Autodesk Inventor part; units mm, degrees
(part 2 of 2)
  line L838 (-99.3571, 77.0912) -> (-99.3571, 73.3912)
  line L839 (-99.3571, 73.3912) -> (-93.3571, 73.3912)
  line L840 (-93.3571, 73.3912) -> (-93.3571, 74.7912)
  line L841 (-91.3571, 74.7912) -> (-91.3571, 73.3912)
  line L842 (-91.3571, 73.3912) -> (-85.3571, 73.3912)
  line L843 (-85.3571, 73.3912) -> (-85.3571, 77.0912)
  line L844 (-85.3571, 77.0912) -> (-86.3571, 77.0912)
  line L845 (-86.3571, 77.0912) -> (-86.3571, 81.0912)
  spline S16 degree 3 poles (-86.3571, 81.0912) (-86.3571, 81.3565) (-86.4624, 81.6108) (-86.6499, 81.7984) knots 0 0 0 0 0.5 0.5 0.5 0.5
  line L846 (-86.3571, 81.0912) -> (-86.3571, 81.3565) construction
  line L847 (-86.3571, 81.3565) -> (-86.4624, 81.6108) construction
  line L848 (-86.4624, 81.6108) -> (-86.6499, 81.7984) construction
  spline S17 degree 3 poles (-86.6499, 81.7984) (-86.6501, 81.7986) (-86.8375, 81.9859) (-87.0918, 82.0912) (-87.3571, 82.0912) knots 0.5 0.5 0.5 0.5 0.5 1 1 1 1
  line L849 (-86.6499, 81.7984) -> (-86.6499, 81.7984) construction
  line L850 (-86.6499, 81.7984) -> (-86.8375, 81.9859) construction
  line L851 (-86.8375, 81.9859) -> (-87.0918, 82.0912) construction
  line L852 (-87.0918, 82.0912) -> (-87.3571, 82.0912) construction
  line L853 (-87.3571, 82.0912) -> (-89.3571, 82.0912)
  spline S18 degree 3 poles (-89.3571, 82.0912) (-89.6223, 82.0912) (-89.8766, 81.9859) (-90.0642, 81.7984) knots 0 0 0 0 0.5 0.5 0.5 0.5
  line L854 (-89.3571, 82.0912) -> (-89.6223, 82.0912) construction
  line L855 (-89.6223, 82.0912) -> (-89.8766, 81.9859) construction
  line L856 (-89.8766, 81.9859) -> (-90.0642, 81.7984) construction
  spline S19 degree 3 poles (-90.0642, 81.7984) (-90.0644, 81.7982) (-90.2517, 81.6108) (-90.3571, 81.3565) (-90.3571, 81.0912) knots 0.5 0.5 0.5 0.5 0.5 1 1 1 1
  line L857 (-90.0642, 81.7984) -> (-90.0642, 81.7984) construction
  line L858 (-90.0642, 81.7984) -> (-90.2517, 81.6108) construction
  line L859 (-90.2517, 81.6108) -> (-90.3571, 81.3565) construction
  line L860 (-90.3571, 81.3565) -> (-90.3571, 81.0912) construction
  line L861 (-90.3571, 81.0912) -> (-90.3571, 77.0912)
  line L862 (-90.3571, 77.0912) -> (-91.3571, 77.0912)
  line L863 (-91.3571, 77.0912) -> (-91.3571, 75.0912)
  line L864 (-91.3571, 91.7912) -> (-91.3571, 90.3912)
  line L865 (-91.3571, 90.3912) -> (-85.3571, 90.3912)
  line L866 (-85.3571, 90.3912) -> (-85.3571, 94.0912)
  line L867 (-85.3571, 94.0912) -> (-86.3571, 94.0912)
  line L868 (-86.3571, 94.0912) -> (-86.3571, 98.0911)
  spline S20 degree 3 poles (-86.3571, 98.0911) (-86.3571, 98.3564) (-86.4624, 98.6107) (-86.6499, 98.7983) knots 0 0 0 0 0.5 0.5 0.5 0.5
  line L869 (-86.3571, 98.0911) -> (-86.3571, 98.3564) construction
  line L870 (-86.3571, 98.3564) -> (-86.4624, 98.6107) construction
  line L871 (-86.4624, 98.6107) -> (-86.6499, 98.7983) construction
  spline S21 degree 3 poles (-86.6499, 98.7983) (-86.6501, 98.7985) (-86.8375, 98.9858) (-87.0918, 99.0911) (-87.3571, 99.0911) knots 0.5 0.5 0.5 0.5 0.5 1 1 1 1
  line L872 (-86.6499, 98.7983) -> (-86.6499, 98.7983) construction
  line L873 (-86.6499, 98.7983) -> (-86.8375, 98.9858) construction
  line L874 (-86.8375, 98.9858) -> (-87.0918, 99.0911) construction
  line L875 (-87.0918, 99.0911) -> (-87.3571, 99.0911) construction
  line L876 (-87.3571, 99.0911) -> (-89.3571, 99.0911)
  spline S22 degree 3 poles (-89.3571, 99.0911) (-89.6223, 99.0911) (-89.8766, 98.9858) (-90.0642, 98.7983) knots 0 0 0 0 0.5 0.5 0.5 0.5
  line L877 (-89.3571, 99.0911) -> (-89.6223, 99.0911) construction
  line L878 (-89.6223, 99.0911) -> (-89.8766, 98.9858) construction
  line L879 (-89.8766, 98.9858) -> (-90.0642, 98.7983) construction
  spline S23 degree 3 poles (-90.0642, 98.7983) (-90.0644, 98.7981) (-90.2517, 98.6107) (-90.3571, 98.3564) (-90.3571, 98.0911) knots 0.5 0.5 0.5 0.5 0.5 1 1 1 1
  line L880 (-90.0642, 98.7983) -> (-90.0642, 98.7983) construction
  line L881 (-90.0642, 98.7983) -> (-90.2517, 98.6107) construction
  line L882 (-90.2517, 98.6107) -> (-90.3571, 98.3564) construction
  line L883 (-90.3571, 98.3564) -> (-90.3571, 98.0911) construction
  line L884 (-90.3571, 98.0911) -> (-90.3571, 94.0912)
  line L885 (-90.3571, 94.0912) -> (-91.3571, 94.0912)
  line L886 (-91.3571, 94.0912) -> (-91.3571, 92.0912)
  line L887 (-93.3571, 92.0912) -> (-93.3571, 94.0912)
  line L888 (-93.3571, 94.0912) -> (-94.3571, 94.0912)
  line L889 (-94.3571, 94.0912) -> (-94.3571, 98.0911)
  spline S24 degree 3 poles (-94.3571, 98.0911) (-94.3571, 98.3564) (-94.4624, 98.6107) (-94.6499, 98.7983) knots 0 0 0 0 0.5 0.5 0.5 0.5
  line L890 (-94.3571, 98.0911) -> (-94.3571, 98.3564) construction
  line L891 (-94.3571, 98.3564) -> (-94.4624, 98.6107) construction
  line L892 (-94.4624, 98.6107) -> (-94.6499, 98.7983) construction
  spline S25 degree 3 poles (-94.6499, 98.7983) (-94.6501, 98.7985) (-94.8375, 98.9858) (-95.0918, 99.0911) (-95.3571, 99.0911) knots 0.5 0.5 0.5 0.5 0.5 1 1 1 1
  line L893 (-94.6499, 98.7983) -> (-94.6499, 98.7983) construction
  line L894 (-94.6499, 98.7983) -> (-94.8375, 98.9858) construction
  line L895 (-94.8375, 98.9858) -> (-95.0918, 99.0911) construction
  line L896 (-95.0918, 99.0911) -> (-95.3571, 99.0911) construction
  line L897 (-95.3571, 99.0911) -> (-97.3571, 99.0911)
  spline S26 degree 3 poles (-97.3571, 99.0911) (-97.6223, 99.0911) (-97.8766, 98.9858) (-98.0642, 98.7983) knots 0 0 0 0 0.5 0.5 0.5 0.5
  line L898 (-97.3571, 99.0911) -> (-97.6223, 99.0911) construction
  line L899 (-97.6223, 99.0911) -> (-97.8766, 98.9858) construction
  line L900 (-97.8766, 98.9858) -> (-98.0642, 98.7983) construction
  spline S27 degree 3 poles (-98.0642, 98.7983) (-98.0644, 98.7981) (-98.2517, 98.6107) (-98.3571, 98.3564) (-98.3571, 98.0911) knots 0.5 0.5 0.5 0.5 0.5 1 1 1 1
  line L901 (-98.0642, 98.7983) -> (-98.0642, 98.7983) construction
  line L902 (-98.0642, 98.7983) -> (-98.2517, 98.6107) construction
  line L903 (-98.2517, 98.6107) -> (-98.3571, 98.3564) construction
  line L904 (-98.3571, 98.3564) -> (-98.3571, 98.0911) construction
  line L905 (-98.3571, 98.0911) -> (-98.3571, 94.0912)
  line L906 (-98.3571, 94.0912) -> (-99.3571, 94.0912)
  line L907 (-99.3571, 94.0912) -> (-99.3571, 90.3912)
  line L908 (-99.3571, 90.3912) -> (-93.3571, 90.3912)
  line L909 (-93.3571, 90.3912) -> (-93.3571, 91.7912)
  line L910 (-93.3571, 91.7912) -> (-91.3571, 91.7912)
  line L911 (-91.3571, 92.0912) -> (-93.3571, 92.0912)
  line L912 (-38.6965, 73.0892) -> (-34.6965, 73.0892)
  line L913 (-34.6965, 73.0892) -> (-34.6965, 76.0892)
  line L914 (-34.6965, 76.0892) -> (-38.6965, 76.0892)
  line L915 (-38.6965, 76.0892) -> (-38.6965, 73.0892)
  line L916 (-93.2175, 103.1942) -> (-89.2175, 103.1942)
  line L917 (-89.2175, 103.1942) -> (-89.2175, 106.1942)
  line L918 (-89.2175, 106.1942) -> (-93.2175, 106.1942)
  line L919 (-93.2175, 106.1942) -> (-93.2175, 103.1942)
  line L920 (-93.2175, 110.1942) -> (-89.2175, 110.1942)
  line L921 (-89.2175, 110.1942) -> (-89.2175, 113.1942)
  line L922 (-89.2175, 113.1942) -> (-93.2175, 113.1942)
  line L923 (-93.2175, 113.1942) -> (-93.2175, 110.1942)
  line L924 (73.6427, 117.4429) -> (68.6427, 117.4429)
  line L925 (68.6427, 117.4429) -> (68.6427, 120.4429)
  line L926 (68.6427, 120.4429) -> (73.6427, 120.4429)
  line L927 (73.6427, 120.4429) -> (73.6427, 117.4429)
  line L928 (73.6427, 58.7395) -> (68.6427, 58.7395)
  line L929 (68.6427, 58.7395) -> (68.6427, 55.7395)
  line L930 (68.6427, 55.7395) -> (73.6427, 55.7395)
  line L931 (73.6427, 55.7395) -> (73.6427, 58.7395)
  line L932 (-93.1735, 117.4429) -> (-88.1735, 117.4429)
  line L933 (-88.1735, 117.4429) -> (-88.1735, 120.4429)
  line L934 (-88.1735, 120.4429) -> (-93.1735, 120.4429)
  line L935 (-93.1735, 120.4429) -> (-93.1735, 117.4429)
  spline S28 degree 3 poles (-84.0914, 112.2529) (-84.0914, 113.0813) (-84.763, 113.7529) (-85.5914, 113.7529) knots 0 0 0 0 0.25 0.25 0.25 0.25
  line L936 (-84.0914, 112.2529) -> (-84.0914, 113.0813) construction
  line L937 (-84.0914, 113.0813) -> (-84.763, 113.7529) construction
  line L938 (-84.763, 113.7529) -> (-85.5914, 113.7529) construction
  line L939 (-85.5914, 113.7529) -> (-85.5914, 113.7529) construction
  line L940 (-85.5914, 113.7529) -> (-86.4199, 113.7529) construction
  line L941 (-86.4199, 113.7529) -> (-87.0914, 113.0813) construction
  line L942 (-87.0914, 113.0813) -> (-87.0914, 112.2529) construction
  line L943 (-87.0914, 112.2529) -> (-87.0914, 112.2529) construction
  line L944 (-87.0914, 112.2529) -> (-87.0914, 111.4245) construction
  line L945 (-87.0914, 111.4245) -> (-86.4199, 110.7529) construction
  line L946 (-86.4199, 110.7529) -> (-85.5914, 110.7529) construction
  line L947 (-85.5914, 110.7529) -> (-85.5914, 110.7529) construction
  line L948 (-85.5914, 110.7529) -> (-84.763, 110.7529) construction
  line L949 (-84.763, 110.7529) -> (-84.0914, 111.4245) construction
  line L950 (-84.0914, 111.4245) -> (-84.0914, 112.2529) construction
  spline S29 degree 3 poles (-84.0914, 63.993) (-84.0914, 64.8214) (-84.763, 65.493) (-85.5914, 65.493) knots 0 0 0 0 0.25 0.25 0.25 0.25
  line L951 (-84.0914, 63.993) -> (-84.0914, 64.8214) construction
  line L952 (-84.0914, 64.8214) -> (-84.763, 65.493) construction
  line L953 (-84.763, 65.493) -> (-85.5914, 65.493) construction
  line L954 (-85.5914, 65.493) -> (-85.5914, 65.493) construction
  line L955 (-85.5914, 65.493) -> (-86.4199, 65.493) construction
  line L956 (-86.4199, 65.493) -> (-87.0914, 64.8214) construction
  line L957 (-87.0914, 64.8214) -> (-87.0914, 63.993) construction
  line L958 (-87.0914, 63.993) -> (-87.0914, 63.993) construction
  line L959 (-87.0914, 63.993) -> (-87.0914, 63.1646) construction
  line L960 (-87.0914, 63.1646) -> (-86.4199, 62.493) construction
  line L961 (-86.4199, 62.493) -> (-85.5914, 62.493) construction
  line L962 (-85.5914, 62.493) -> (-85.5914, 62.493) construction
  line L963 (-85.5914, 62.493) -> (-84.763, 62.493) construction
  line L964 (-84.763, 62.493) -> (-84.0914, 63.1646) construction
  line L965 (-84.0914, 63.1646) -> (-84.0914, 63.993) construction
  spline S30 degree 3 poles (-18.0514, 67.168) (-18.0514, 67.9964) (-18.723, 68.668) (-19.5514, 68.668) knots 0 0 0 0 0.25 0.25 0.25 0.25
  line L966 (-18.0514, 67.168) -> (-18.0514, 67.9964) construction
  line L967 (-18.0514, 67.9964) -> (-18.723, 68.668) construction
  line L968 (-18.723, 68.668) -> (-19.5514, 68.668) construction
  line L969 (-19.5514, 68.668) -> (-19.5514, 68.668) construction
  line L970 (-19.5514, 68.668) -> (-20.3799, 68.668) construction
  line L971 (-20.3799, 68.668) -> (-21.0514, 67.9964) construction
  line L972 (-21.0514, 67.9964) -> (-21.0514, 67.168) construction
  line L973 (-21.0514, 67.168) -> (-21.0514, 67.168) construction
  line L974 (-21.0514, 67.168) -> (-21.0514, 66.3396) construction
  line L975 (-21.0514, 66.3396) -> (-20.3799, 65.668) construction
  line L976 (-20.3799, 65.668) -> (-19.5514, 65.668) construction
  line L977 (-19.5514, 65.668) -> (-19.5514, 65.668) construction
  line L978 (-19.5514, 65.668) -> (-18.723, 65.668) construction
  line L979 (-18.723, 65.668) -> (-18.0514, 66.3396) construction
  line L980 (-18.0514, 66.3396) -> (-18.0514, 67.168) construction
  line L981 (-100.3571, 66.5242) -> (-100.3571, 55.7396)
  line L982 (-100.3571, 55.7395) -> (-100.3553, 55.6371)
  line L983 (-100.3553, 55.6371) -> (-100.3501, 55.5348)
  line L984 (-100.3501, 55.5348) -> (-100.3413, 55.4327)
  line L985 (-100.3413, 55.4327) -> (-100.3291, 55.331)
  line L986 (-100.3291, 55.331) -> (-100.3134, 55.2298)
  line L987 (-100.3134, 55.2298) -> (-100.2943, 55.1291)
  line L988 (-100.2943, 55.1291) -> (-100.2718, 55.0292)
  line L989 (-100.2718, 55.0292) -> (-100.2458, 54.9301)
  line L990 (-100.2458, 54.9301) -> (-100.2165, 54.832)
  line L991 (-100.2165, 54.832) -> (-100.1838, 54.7349)
  line L992 (-100.1838, 54.7349) -> (-100.1479, 54.6389)
  line L993 (-100.1479, 54.6389) -> (-100.1087, 54.5443)
  line L994 (-100.1087, 54.5443) -> (-100.0663, 54.451)
  line L995 (-100.0663, 54.451) -> (-100.0207, 54.3593)
  line L996 (-100.0207, 54.3593) -> (-99.972, 54.2692)
  line L997 (-99.972, 54.2692) -> (-99.9203, 54.1807)
  line L998 (-99.9203, 54.1807) -> (-99.8656, 54.0941)
  line L999 (-99.8656, 54.0941) -> (-99.808, 54.0095)
  line L1000 (-99.808, 54.0095) -> (-99.7475, 53.9268)
  line L1001 (-99.7475, 53.9268) -> (-99.6842, 53.8462)
  line L1002 (-99.6842, 53.8462) -> (-99.6182, 53.7679)
  line L1003 (-99.6182, 53.7679) -> (-99.5496, 53.6918)
  line L1004 (-99.5496, 53.6918) -> (-99.4784, 53.6182)
  line L1005 (-99.4784, 53.6182) -> (-99.4047, 53.547)
  line L1006 (-99.4047, 53.547) -> (-99.3287, 53.4784)
  line L1007 (-99.3287, 53.4784) -> (-99.2503, 53.4124)
  line L1008 (-99.2503, 53.4124) -> (-99.1698, 53.3491)
  line L1009 (-99.1698, 53.3491) -> (-99.0871, 53.2886)
  line L1010 (-99.0871, 53.2886) -> (-99.0024, 53.231)
  line L1011 (-99.0024, 53.231) -> (-98.9158, 53.1762)
  line L1012 (-98.9158, 53.1762) -> (-98.8274, 53.1245)
  line L1013 (-98.8274, 53.1245) -> (-98.7372, 53.0758)
  line L1014 (-98.7372, 53.0758) -> (-98.6455, 53.0303)
  line L1015 (-98.6455, 53.0303) -> (-98.5523, 52.9879)
  line L1016 (-98.5523, 52.9879) -> (-98.4576, 52.9487)
  line L1017 (-98.4576, 52.9487) -> (-98.3617, 52.9127)
  line L1018 (-98.3617, 52.9127) -> (-98.2646, 52.8801)
  line L1019 (-98.2646, 52.8801) -> (-98.1664, 52.8507)
  line L1020 (-98.1664, 52.8507) -> (-98.0673, 52.8248)
  line L1021 (-98.0673, 52.8248) -> (-97.9674, 52.8022)
  line L1022 (-97.9674, 52.8022) -> (-97.8668, 52.7831)
  line L1023 (-97.8668, 52.7831) -> (-97.7655, 52.7674)
  line L1024 (-97.7655, 52.7674) -> (-97.6638, 52.7552)
  line L1025 (-97.6638, 52.7552) -> (-97.5618, 52.7465)
  line L1026 (-97.5618, 52.7465) -> (-97.4595, 52.7412)
  line L1027 (-97.4595, 52.7412) -> (-97.3571, 52.7395)
  line L1028 (-97.3571, 52.7395) -> (-16.3571, 52.7395)
  line L1029 (-16.3571, 52.7395) -> (-16.2546, 52.7412)
  line L1030 (-16.2546, 52.7412) -> (-16.1523, 52.7465)
  line L1031 (-16.1523, 52.7465) -> (-16.0503, 52.7552)
  line L1032 (-16.0503, 52.7552) -> (-15.9486, 52.7674)
  line L1033 (-15.9486, 52.7674) -> (-15.8473, 52.7831)
  line L1034 (-15.8473, 52.7831) -> (-15.7467, 52.8022)
  line L1035 (-15.7467, 52.8022) -> (-15.6468, 52.8248)
  line L1036 (-15.6468, 52.8248) -> (-15.5477, 52.8507)
  line L1037 (-15.5477, 52.8507) -> (-15.4495, 52.8801)
  line L1038 (-15.4495, 52.8801) -> (-15.3524, 52.9127)
  line L1039 (-15.3524, 52.9127) -> (-15.2565, 52.9487)
  line L1040 (-15.2565, 52.9487) -> (-15.1618, 52.9879)
  line L1041 (-15.1618, 52.9879) -> (-15.0686, 53.0303)
  line L1042 (-15.0686, 53.0303) -> (-14.9769, 53.0758)
  line L1043 (-14.9769, 53.0758) -> (-14.8867, 53.1245)
  line L1044 (-14.8867, 53.1245) -> (-14.7983, 53.1762)
  line L1045 (-14.7983, 53.1762) -> (-14.7117, 53.231)
  line L1046 (-14.7117, 53.231) -> (-14.627, 53.2886)
  line L1047 (-14.627, 53.2886) -> (-14.5443, 53.3491)
  line L1048 (-14.5443, 53.3491) -> (-14.4638, 53.4124)
  line L1049 (-14.4638, 53.4124) -> (-14.3854, 53.4784)
  line L1050 (-14.3854, 53.4784) -> (-14.3094, 53.547)
  line L1051 (-14.3094, 53.547) -> (-14.2357, 53.6182)
  line L1052 (-14.2357, 53.6182) -> (-14.1645, 53.6918)
  line L1053 (-14.1645, 53.6918) -> (-14.0959, 53.7679)
  line L1054 (-14.0959, 53.7679) -> (-14.0299, 53.8462)
  line L1055 (-14.0299, 53.8462) -> (-13.9666, 53.9268)
  line L1056 (-13.9666, 53.9268) -> (-13.9061, 54.0095)
  line L1057 (-13.9061, 54.0095) -> (-13.8485, 54.0941)
  line L1058 (-13.8485, 54.0941) -> (-13.7938, 54.1807)
  line L1059 (-13.7938, 54.1807) -> (-13.7421, 54.2692)
  line L1060 (-13.7421, 54.2692) -> (-13.6934, 54.3593)
  line L1061 (-13.6934, 54.3593) -> (-13.6478, 54.451)
  line L1062 (-13.6478, 54.451) -> (-13.6054, 54.5443)
  line L1063 (-13.6054, 54.5443) -> (-13.5662, 54.6389)
  line L1064 (-13.5662, 54.6389) -> (-13.5303, 54.7349)
  line L1065 (-13.5303, 54.7349) -> (-13.4976, 54.832)
  line L1066 (-13.4976, 54.832) -> (-13.4683, 54.9301)
  line L1067 (-13.4683, 54.9301) -> (-13.4423, 55.0292)
  line L1068 (-13.4423, 55.0292) -> (-13.4198, 55.1291)
  line L1069 (-13.4198, 55.1291) -> (-13.4007, 55.2298)
  line L1070 (-13.4007, 55.2298) -> (-13.385, 55.331)
  line L1071 (-13.385, 55.331) -> (-13.3728, 55.4327)
  line L1072 (-13.3728, 55.4327) -> (-13.364, 55.5348)
  line L1073 (-13.364, 55.5348) -> (-13.3588, 55.6371)
  line L1074 (-13.3588, 55.6371) -> (-13.3571, 55.7395)
  line L1075 (-13.3571, 55.7395) -> (-13.3571, 120.4429)
  line L1076 (-13.3571, 120.4429) -> (-13.3588, 120.5453)
  line L1077 (-13.3588, 120.5453) -> (-13.364, 120.6476)
  line L1078 (-13.364, 120.6476) -> (-13.3728, 120.7497)
  line L1079 (-13.3728, 120.7497) -> (-13.385, 120.8514)
  line L1080 (-13.385, 120.8514) -> (-13.4007, 120.9526)
  line L1081 (-13.4007, 120.9526) -> (-13.4198, 121.0533)
  line L1082 (-13.4198, 121.0533) -> (-13.4423, 121.1532)
  line L1083 (-13.4423, 121.1532) -> (-13.4683, 121.2523)
  line L1084 (-13.4683, 121.2523) -> (-13.4976, 121.3504)
  line L1085 (-13.4976, 121.3504) -> (-13.5303, 121.4475)
  line L1086 (-13.5303, 121.4475) -> (-13.5662, 121.5435)
  line L1087 (-13.5662, 121.5435) -> (-13.6054, 121.6381)
  line L1088 (-13.6054, 121.6381) -> (-13.6478, 121.7314)
  line L1089 (-13.6478, 121.7314) -> (-13.6934, 121.8231)
  line L1090 (-13.6934, 121.8231) -> (-13.7421, 121.9132)
  line L1091 (-13.7421, 121.9132) -> (-13.7938, 122.0017)
  line L1092 (-13.7938, 122.0017) -> (-13.8485, 122.0883)
  line L1093 (-13.8485, 122.0883) -> (-13.9061, 122.1729)
  line L1094 (-13.9061, 122.1729) -> (-13.9666, 122.2556)
  line L1095 (-13.9666, 122.2556) -> (-14.0299, 122.3362)
  line L1096 (-14.0299, 122.3362) -> (-14.0959, 122.4145)
  line L1097 (-14.0959, 122.4145) -> (-14.1645, 122.4906)
  line L1098 (-14.1645, 122.4906) -> (-14.2357, 122.5642)
  line L1099 (-14.2357, 122.5642) -> (-14.3094, 122.6354)
  line L1100 (-14.3094, 122.6354) -> (-14.3854, 122.704)
  line L1101 (-14.3854, 122.704) -> (-14.4638, 122.77)
  line L1102 (-14.4638, 122.77) -> (-14.5443, 122.8333)
  line L1103 (-14.5443, 122.8333) -> (-14.627, 122.8938)
  line L1104 (-14.627, 122.8938) -> (-14.7117, 122.9514)
  line L1105 (-14.7117, 122.9514) -> (-14.7983, 123.0062)
  line L1106 (-14.7983, 123.0062) -> (-14.8867, 123.0579)
  line L1107 (-14.8867, 123.0579) -> (-14.9769, 123.1066)
  line L1108 (-14.9769, 123.1066) -> (-15.0686, 123.1521)
  line L1109 (-15.0686, 123.1521) -> (-15.1618, 123.1945)
  line L1110 (-15.1618, 123.1945) -> (-15.2565, 123.2337)
  line L1111 (-15.2565, 123.2337) -> (-15.3524, 123.2697)
  line L1112 (-15.3524, 123.2697) -> (-15.4495, 123.3023)
  line L1113 (-15.4495, 123.3023) -> (-15.5477, 123.3317)
  line L1114 (-15.5477, 123.3317) -> (-15.6468, 123.3576)
  line L1115 (-15.6468, 123.3576) -> (-15.7467, 123.3802)
  line L1116 (-15.7467, 123.3802) -> (-15.8473, 123.3993)
  line L1117 (-15.8473, 123.3993) -> (-15.9486, 123.415)
  line L1118 (-15.9486, 123.415) -> (-16.0503, 123.4272)
  line L1119 (-16.0503, 123.4272) -> (-16.1523, 123.4359)
  line L1120 (-16.1523, 123.4359) -> (-16.2546, 123.4412)
  line L1121 (-16.2546, 123.4412) -> (-16.3571, 123.4429)
  line L1122 (-16.3571, 123.4429) -> (-97.3571, 123.4429)
  line L1123 (-97.3571, 123.4429) -> (-97.4595, 123.4412)
  line L1124 (-97.4595, 123.4412) -> (-97.5618, 123.4359)
  line L1125 (-97.5618, 123.4359) -> (-97.6638, 123.4272)
  line L1126 (-97.6638, 123.4272) -> (-97.7655, 123.415)
  line L1127 (-97.7655, 123.415) -> (-97.8668, 123.3993)
  line L1128 (-97.8668, 123.3993) -> (-97.9674, 123.3802)
  line L1129 (-97.9674, 123.3802) -> (-98.0673, 123.3576)
  line L1130 (-98.0673, 123.3576) -> (-98.1664, 123.3317)
  line L1131 (-98.1664, 123.3317) -> (-98.2646, 123.3023)
  line L1132 (-98.2646, 123.3023) -> (-98.3617, 123.2697)
  line L1133 (-98.3617, 123.2697) -> (-98.4576, 123.2337)
  line L1134 (-98.4576, 123.2337) -> (-98.5523, 123.1945)
  line L1135 (-98.5523, 123.1945) -> (-98.6455, 123.1521)
  line L1136 (-98.6455, 123.1521) -> (-98.7372, 123.1066)
  line L1137 (-98.7372, 123.1066) -> (-98.8274, 123.0579)
  line L1138 (-98.8274, 123.0579) -> (-98.9158, 123.0062)
  line L1139 (-98.9158, 123.0062) -> (-99.0024, 122.9514)
  line L1140 (-99.0024, 122.9514) -> (-99.0871, 122.8938)
  line L1141 (-99.0871, 122.8938) -> (-99.1698, 122.8333)
  line L1142 (-99.1698, 122.8333) -> (-99.2503, 122.77)
  line L1143 (-99.2503, 122.77) -> (-99.3287, 122.704)
  line L1144 (-99.3287, 122.704) -> (-99.4047, 122.6354)
  line L1145 (-99.4047, 122.6354) -> (-99.4784, 122.5642)
  line L1146 (-99.4784, 122.5642) -> (-99.5496, 122.4906)
  line L1147 (-99.5496, 122.4906) -> (-99.6182, 122.4145)
  line L1148 (-99.6182, 122.4145) -> (-99.6842, 122.3362)
  line L1149 (-99.6842, 122.3362) -> (-99.7475, 122.2556)
  line L1150 (-99.7475, 122.2556) -> (-99.808, 122.1729)
  line L1151 (-99.808, 122.1729) -> (-99.8656, 122.0883)
  line L1152 (-99.8656, 122.0883) -> (-99.9203, 122.0017)
  line L1153 (-99.9203, 122.0017) -> (-99.972, 121.9132)
  line L1154 (-99.972, 121.9132) -> (-100.0207, 121.8231)
  line L1155 (-100.0207, 121.8231) -> (-100.0663, 121.7314)
  line L1156 (-100.0663, 121.7314) -> (-100.1087, 121.6381)
  line L1157 (-100.1087, 121.6381) -> (-100.1479, 121.5435)
  line L1158 (-100.1479, 121.5435) -> (-100.1838, 121.4475)
  line L1159 (-100.1838, 121.4475) -> (-100.2165, 121.3504)
  line L1160 (-100.2165, 121.3504) -> (-100.2458, 121.2523)
  line L1161 (-100.2458, 121.2523) -> (-100.2718, 121.1532)
  line L1162 (-100.2718, 121.1532) -> (-100.2943, 121.0533)
  line L1163 (-100.2943, 121.0533) -> (-100.3134, 120.9526)
  line L1164 (-100.3134, 120.9526) -> (-100.3291, 120.8514)
  line L1165 (-100.3291, 120.8514) -> (-100.3413, 120.7497)
  line L1166 (-100.3413, 120.7497) -> (-100.3501, 120.6476)
  line L1167 (-100.3501, 120.6476) -> (-100.3553, 120.5453)
  line L1168 (-100.3553, 120.5453) -> (-100.3571, 120.4429)
  line L1169 (-100.3571, 120.4429) -> (-100.3571, 101.0912)
  line L1170 (-3.1737, 58.7395) -> (1.8263, 58.7395)
  line L1171 (1.8263, 58.7395) -> (1.8263, 55.7395)
  line L1172 (1.8263, 55.7395) -> (-3.1737, 55.7395)
  line L1173 (-3.1737, 55.7395) -> (-3.1737, 58.7395)
  line L1174 (76.6427, 55.7395) -> (76.6427, 120.4429)
  line L1175 (76.6427, 120.4429) -> (76.641, 120.5453)
  line L1176 (76.641, 120.5453) -> (76.6358, 120.6476)
  line L1177 (76.6358, 120.6476) -> (76.627, 120.7497)
  line L1178 (76.627, 120.7497) -> (76.6148, 120.8514)
  line L1179 (76.6148, 120.8514) -> (76.5991, 120.9526)
  line L1180 (76.5991, 120.9526) -> (76.58, 121.0533)
  line L1181 (76.58, 121.0533) -> (76.5575, 121.1532)
  line L1182 (76.5575, 121.1532) -> (76.5315, 121.2523)
  line L1183 (76.5315, 121.2523) -> (76.5022, 121.3504)
  line L1184 (76.5022, 121.3504) -> (76.4695, 121.4475)
  line L1185 (76.4695, 121.4475) -> (76.4336, 121.5435)
  line L1186 (76.4336, 121.5435) -> (76.3944, 121.6381)
  line L1187 (76.3944, 121.6381) -> (76.352, 121.7314)
  line L1188 (76.352, 121.7314) -> (76.3064, 121.8231)
  line L1189 (76.3064, 121.8231) -> (76.2577, 121.9132)
  line L1190 (76.2577, 121.9132) -> (76.206, 122.0017)
  line L1191 (76.206, 122.0017) -> (76.1513, 122.0883)
  line L1192 (76.1513, 122.0883) -> (76.0937, 122.1729)
  line L1193 (76.0937, 122.1729) -> (76.0332, 122.2556)
  line L1194 (76.0332, 122.2556) -> (75.9699, 122.3362)
  line L1195 (75.9699, 122.3362) -> (75.9039, 122.4145)
  line L1196 (75.9039, 122.4145) -> (75.8353, 122.4906)
  line L1197 (75.8353, 122.4906) -> (75.7641, 122.5642)
  line L1198 (75.7641, 122.5642) -> (75.6904, 122.6354)
  line L1199 (75.6904, 122.6354) -> (75.6144, 122.704)
  line L1200 (75.6144, 122.704) -> (75.536, 122.77)
  line L1201 (75.536, 122.77) -> (75.4555, 122.8333)
  line L1202 (75.4555, 122.8333) -> (75.3728, 122.8938)
  line L1203 (75.3728, 122.8938) -> (75.2881, 122.9514)
  line L1204 (75.2881, 122.9514) -> (75.2015, 123.0062)
  line L1205 (75.2015, 123.0062) -> (75.1131, 123.0579)
  line L1206 (75.1131, 123.0579) -> (75.0229, 123.1066)
  line L1207 (75.0229, 123.1066) -> (74.9312, 123.1521)
  line L1208 (74.9312, 123.1521) -> (74.838, 123.1945)
  line L1209 (74.838, 123.1945) -> (74.7433, 123.2337)
  line L1210 (74.7433, 123.2337) -> (74.6474, 123.2697)
  line L1211 (74.6474, 123.2697) -> (74.5503, 123.3023)
  line L1212 (74.5503, 123.3023) -> (74.4521, 123.3317)
  line L1213 (74.4521, 123.3317) -> (74.353, 123.3576)
  line L1214 (74.353, 123.3576) -> (74.2531, 123.3802)
  line L1215 (74.2531, 123.3802) -> (74.1525, 123.3993)
  line L1216 (74.1525, 123.3993) -> (74.0512, 123.415)
  line L1217 (74.0512, 123.415) -> (73.9495, 123.4272)
  line L1218 (73.9495, 123.4272) -> (73.8475, 123.4359)
  line L1219 (73.8475, 123.4359) -> (73.7452, 123.4412)
  line L1220 (73.7452, 123.4412) -> (73.6427, 123.4429)
  line L1221 (73.6427, 123.4429) -> (-7.3572, 123.4429)
  line L1222 (-7.3572, 123.4429) -> (-7.4596, 123.4412)
  line L1223 (-7.4596, 123.4412) -> (-7.5619, 123.4359)
  line L1224 (-7.5619, 123.4359) -> (-7.6639, 123.4272)
  line L1225 (-7.6639, 123.4272) -> (-7.7656, 123.415)
  line L1226 (-7.7656, 123.415) -> (-7.8669, 123.3993)
  line L1227 (-7.8669, 123.3993) -> (-7.9675, 123.3802)
  line L1228 (-7.9675, 123.3802) -> (-8.0674, 123.3576)
  line L1229 (-8.0674, 123.3576) -> (-8.1665, 123.3317)
  line L1230 (-8.1665, 123.3317) -> (-8.2647, 123.3023)
  line L1231 (-8.2647, 123.3023) -> (-8.3618, 123.2697)
  line L1232 (-8.3618, 123.2697) -> (-8.4577, 123.2337)
  line L1233 (-8.4577, 123.2337) -> (-8.5524, 123.1945)
  line L1234 (-8.5524, 123.1945) -> (-8.6456, 123.1521)
  line L1235 (-8.6456, 123.1521) -> (-8.7373, 123.1066)
  line L1236 (-8.7373, 123.1066) -> (-8.8275, 123.0579)
  line L1237 (-8.8275, 123.0579) -> (-8.9159, 123.0062)
  line L1238 (-8.9159, 123.0062) -> (-9.0025, 122.9514)
  line L1239 (-9.0025, 122.9514) -> (-9.0872, 122.8938)
  line L1240 (-9.0872, 122.8938) -> (-9.1699, 122.8333)
  line L1241 (-9.1699, 122.8333) -> (-9.2504, 122.77)
  line L1242 (-9.2504, 122.77) -> (-9.3288, 122.704)
  line L1243 (-9.3288, 122.704) -> (-9.4048, 122.6354)
  line L1244 (-9.4048, 122.6354) -> (-9.4785, 122.5642)
  line L1245 (-9.4785, 122.5642) -> (-9.5497, 122.4906)
  line L1246 (-9.5497, 122.4906) -> (-9.6183, 122.4145)
  line L1247 (-9.6183, 122.4145) -> (-9.6843, 122.3362)
  line L1248 (-9.6843, 122.3362) -> (-9.7476, 122.2556)
  line L1249 (-9.7476, 122.2556) -> (-9.8081, 122.1729)
  line L1250 (-9.8081, 122.1729) -> (-9.8657, 122.0883)
  line L1251 (-9.8657, 122.0883) -> (-9.9204, 122.0017)
  line L1252 (-9.9204, 122.0017) -> (-9.9721, 121.9132)
  line L1253 (-9.9721, 121.9132) -> (-10.0208, 121.8231)
  line L1254 (-10.0208, 121.8231) -> (-10.0664, 121.7314)
  line L1255 (-10.0664, 121.7314) -> (-10.1088, 121.6381)
  line L1256 (-10.1088, 121.6381) -> (-10.148, 121.5435)
  line L1257 (-10.148, 121.5435) -> (-10.1839, 121.4475)
  line L1258 (-10.1839, 121.4475) -> (-10.2166, 121.3504)
  line L1259 (-10.2166, 121.3504) -> (-10.2459, 121.2523)
  line L1260 (-10.2459, 121.2523) -> (-10.2719, 121.1532)
  line L1261 (-10.2719, 121.1532) -> (-10.2944, 121.0533)
  line L1262 (-10.2944, 121.0533) -> (-10.3135, 120.9526)
  line L1263 (-10.3135, 120.9526) -> (-10.3292, 120.8514)
  line L1264 (-10.3292, 120.8514) -> (-10.3414, 120.7497)
  line L1265 (-10.3414, 120.7497) -> (-10.3502, 120.6476)
  line L1266 (-10.3502, 120.6476) -> (-10.3554, 120.5453)
  line L1267 (-10.3554, 120.5453) -> (-10.3572, 120.4429)
  line L1268 (-10.3572, 120.4429) -> (-10.3572, 55.7395)
  line L1269 (-10.3572, 55.7395) -> (-10.3554, 55.6371)
  line L1270 (-10.3554, 55.6371) -> (-10.3502, 55.5348)
  line L1271 (-10.3502, 55.5348) -> (-10.3414, 55.4327)
  line L1272 (-10.3414, 55.4327) -> (-10.3292, 55.331)
  line L1273 (-10.3292, 55.331) -> (-10.3135, 55.2298)
  line L1274 (-10.3135, 55.2298) -> (-10.2944, 55.1291)
  line L1275 (-10.2944, 55.1291) -> (-10.2719, 55.0292)
  line L1276 (-10.2719, 55.0292) -> (-10.2459, 54.9301)
  line L1277 (-10.2459, 54.9301) -> (-10.2166, 54.832)
  line L1278 (-10.2166, 54.832) -> (-10.1839, 54.7349)
  line L1279 (-10.1839, 54.7349) -> (-10.148, 54.6389)
  line L1280 (-10.148, 54.6389) -> (-10.1088, 54.5443)
  line L1281 (-10.1088, 54.5443) -> (-10.0664, 54.451)
  line L1282 (-10.0664, 54.451) -> (-10.0208, 54.3593)
  line L1283 (-10.0208, 54.3593) -> (-9.9721, 54.2692)
  line L1284 (-9.9721, 54.2692) -> (-9.9204, 54.1807)
  line L1285 (-9.9204, 54.1807) -> (-9.8657, 54.0941)
  line L1286 (-9.8657, 54.0941) -> (-9.8081, 54.0095)
  line L1287 (-9.8081, 54.0095) -> (-9.7476, 53.9268)
  line L1288 (-9.7476, 53.9268) -> (-9.6843, 53.8462)
  line L1289 (-9.6843, 53.8462) -> (-9.6183, 53.7679)
  line L1290 (-9.6183, 53.7679) -> (-9.5497, 53.6918)
  line L1291 (-9.5497, 53.6918) -> (-9.4785, 53.6182)
  line L1292 (-9.4785, 53.6182) -> (-9.4048, 53.547)
  line L1293 (-9.4048, 53.547) -> (-9.3288, 53.4784)
  line L1294 (-9.3288, 53.4784) -> (-9.2504, 53.4124)
  line L1295 (-9.2504, 53.4124) -> (-9.1699, 53.3491)
  line L1296 (-9.1699, 53.3491) -> (-9.0872, 53.2886)
  line L1297 (-9.0872, 53.2886) -> (-9.0025, 53.231)
  line L1298 (-9.0025, 53.231) -> (-8.9159, 53.1762)
  line L1299 (-8.9159, 53.1762) -> (-8.8275, 53.1245)
  line L1300 (-8.8275, 53.1245) -> (-8.7373, 53.0758)
  line L1301 (-8.7373, 53.0758) -> (-8.6456, 53.0303)
  line L1302 (-8.6456, 53.0303) -> (-8.5524, 52.9879)
  line L1303 (-8.5524, 52.9879) -> (-8.4577, 52.9487)
  line L1304 (-8.4577, 52.9487) -> (-8.3618, 52.9127)
  line L1305 (-8.3618, 52.9127) -> (-8.2647, 52.8801)
  line L1306 (-8.2647, 52.8801) -> (-8.1665, 52.8507)
  line L1307 (-8.1665, 52.8507) -> (-8.0674, 52.8248)
  line L1308 (-8.0674, 52.8248) -> (-7.9675, 52.8022)
  line L1309 (-7.9675, 52.8022) -> (-7.8669, 52.7831)
  line L1310 (-7.8669, 52.7831) -> (-7.7656, 52.7674)
  line L1311 (-7.7656, 52.7674) -> (-7.6639, 52.7552)
  line L1312 (-7.6639, 52.7552) -> (-7.5619, 52.7465)
  line L1313 (-7.5619, 52.7465) -> (-7.4596, 52.7412)
  line L1314 (-7.4596, 52.7412) -> (-7.3572, 52.7395)
  line L1315 (-7.3572, 52.7395) -> (73.6427, 52.7395)
  line L1316 (73.6427, 52.7395) -> (73.7452, 52.7412)
  line L1317 (73.7452, 52.7412) -> (73.8475, 52.7465)
  line L1318 (73.8475, 52.7465) -> (73.9495, 52.7552)
  line L1319 (73.9495, 52.7552) -> (74.0512, 52.7674)
  line L1320 (74.0512, 52.7674) -> (74.1525, 52.7831)
  line L1321 (74.1525, 52.7831) -> (74.2531, 52.8022)
  line L1322 (74.2531, 52.8022) -> (74.353, 52.8248)
  line L1323 (74.353, 52.8248) -> (74.4521, 52.8507)
  line L1324 (74.4521, 52.8507) -> (74.5503, 52.8801)
  line L1325 (74.5503, 52.8801) -> (74.6474, 52.9127)
  line L1326 (74.6474, 52.9127) -> (74.7433, 52.9487)
  line L1327 (74.7433, 52.9487) -> (74.838, 52.9879)
  line L1328 (74.838, 52.9879) -> (74.9312, 53.0303)
  line L1329 (74.9312, 53.0303) -> (75.0229, 53.0758)
  line L1330 (75.0229, 53.0758) -> (75.1131, 53.1245)
  line L1331 (75.1131, 53.1245) -> (75.2015, 53.1762)
  line L1332 (75.2015, 53.1762) -> (75.2881, 53.231)
  line L1333 (75.2881, 53.231) -> (75.3728, 53.2886)
  line L1334 (75.3728, 53.2886) -> (75.4555, 53.3491)
  line L1335 (75.4555, 53.3491) -> (75.536, 53.4124)
  line L1336 (75.536, 53.4124) -> (75.6144, 53.4784)
  line L1337 (75.6144, 53.4784) -> (75.6904, 53.547)
  line L1338 (75.6904, 53.547) -> (75.7641, 53.6182)
  line L1339 (75.7641, 53.6182) -> (75.8353, 53.6918)
  line L1340 (75.8353, 53.6918) -> (75.9039, 53.7679)
  line L1341 (75.9039, 53.7679) -> (75.9699, 53.8462)
  line L1342 (75.9699, 53.8462) -> (76.0332, 53.9268)
  line L1343 (76.0332, 53.9268) -> (76.0937, 54.0095)
  line L1344 (76.0937, 54.0095) -> (76.1513, 54.0941)
  line L1345 (76.1513, 54.0941) -> (76.206, 54.1807)
  line L1346 (76.206, 54.1807) -> (76.2577, 54.2692)
  line L1347 (76.2577, 54.2692) -> (76.3064, 54.3593)
  line L1348 (76.3064, 54.3593) -> (76.352, 54.451)
  line L1349 (76.352, 54.451) -> (76.3944, 54.5443)
  line L1350 (76.3944, 54.5443) -> (76.4336, 54.6389)
  line L1351 (76.4336, 54.6389) -> (76.4695, 54.7349)
  line L1352 (76.4695, 54.7349) -> (76.5022, 54.832)
  line L1353 (76.5022, 54.832) -> (76.5315, 54.9301)
  line L1354 (76.5315, 54.9301) -> (76.5575, 55.0292)
  line L1355 (76.5575, 55.0292) -> (76.58, 55.1291)
  line L1356 (76.58, 55.1291) -> (76.5991, 55.2298)
  line L1357 (76.5991, 55.2298) -> (76.6148, 55.331)
  line L1358 (76.6148, 55.331) -> (76.627, 55.4327)
  line L1359 (76.627, 55.4327) -> (76.6358, 55.5348)
  line L1360 (76.6358, 55.5348) -> (76.641, 55.6371)
  line L1361 (76.641, 55.6371) -> (76.6427, 55.7395)
  spline S31 degree 3 poles (71.9484, 67.168) (71.9484, 67.9964) (71.2768, 68.668) (70.4484, 68.668) knots 0 0 0 0 0.25 0.25 0.25 0.25
  line L1362 (71.9484, 67.168) -> (71.9484, 67.9964) construction
  line L1363 (71.9484, 67.9964) -> (71.2768, 68.668) construction
  line L1364 (71.2768, 68.668) -> (70.4484, 68.668) construction
  line L1365 (70.4484, 68.668) -> (70.4484, 68.668) construction
  line L1366 (70.4484, 68.668) -> (69.6199, 68.668) construction
  line L1367 (69.6199, 68.668) -> (68.9484, 67.9964) construction
  line L1368 (68.9484, 67.9964) -> (68.9484, 67.168) construction
  line L1369 (68.9484, 67.168) -> (68.9484, 67.168) construction
  line L1370 (68.9484, 67.168) -> (68.9484, 66.3396) construction
  line L1371 (68.9484, 66.3396) -> (69.6199, 65.668) construction
  line L1372 (69.6199, 65.668) -> (70.4484, 65.668) construction
  line L1373 (70.4484, 65.668) -> (70.4484, 65.668) construction
  line L1374 (70.4484, 65.668) -> (71.2768, 65.668) construction
  line L1375 (71.2768, 65.668) -> (71.9484, 66.3396) construction
  line L1376 (71.9484, 66.3396) -> (71.9484, 67.168) construction
  spline S32 degree 3 poles (5.9084, 63.993) (5.9084, 64.8214) (5.2368, 65.493) (4.4084, 65.493) knots 0 0 0 0 0.25 0.25 0.25 0.25
  line L1377 (5.9084, 63.993) -> (5.9084, 64.8214) construction
  line L1378 (5.9084, 64.8214) -> (5.2368, 65.493) construction
  line L1379 (5.2368, 65.493) -> (4.4084, 65.493) construction
  line L1380 (4.4084, 65.493) -> (4.4084, 65.493) construction
  line L1381 (4.4084, 65.493) -> (3.5799, 65.493) construction
  line L1382 (3.5799, 65.493) -> (2.9084, 64.8214) construction
  line L1383 (2.9084, 64.8214) -> (2.9084, 63.993) construction
  line L1384 (2.9084, 63.993) -> (2.9084, 63.993) construction
  line L1385 (2.9084, 63.993) -> (2.9084, 63.1646) construction
  line L1386 (2.9084, 63.1646) -> (3.5799, 62.493) construction
  line L1387 (3.5799, 62.493) -> (4.4084, 62.493) construction
  line L1388 (4.4084, 62.493) -> (4.4084, 62.493) construction
  line L1389 (4.4084, 62.493) -> (5.2368, 62.493) construction
  line L1390 (5.2368, 62.493) -> (5.9084, 63.1646) construction
  line L1391 (5.9084, 63.1646) -> (5.9084, 63.993) construction
  spline S33 degree 3 poles (5.9084, 112.2529) (5.9084, 113.0813) (5.2368, 113.7529) (4.4084, 113.7529) knots 0 0 0 0 0.25 0.25 0.25 0.25
  line L1392 (5.9084, 112.2529) -> (5.9084, 113.0813) construction
  line L1393 (5.9084, 113.0813) -> (5.2368, 113.7529) construction
  line L1394 (5.2368, 113.7529) -> (4.4084, 113.7529) construction
  line L1395 (4.4084, 113.7529) -> (4.4084, 113.7529) construction
  line L1396 (4.4084, 113.7529) -> (3.5799, 113.7529) construction
  line L1397 (3.5799, 113.7529) -> (2.9084, 113.0813) construction
  line L1398 (2.9084, 113.0813) -> (2.9084, 112.2529) construction
  line L1399 (2.9084, 112.2529) -> (2.9084, 112.2529) construction
  line L1400 (2.9084, 112.2529) -> (2.9084, 111.4245) construction
  line L1401 (2.9084, 111.4245) -> (3.5799, 110.7529) construction
  line L1402 (3.5799, 110.7529) -> (4.4084, 110.7529) construction
  line L1403 (4.4084, 110.7529) -> (4.4084, 110.7529) construction
  line L1404 (4.4084, 110.7529) -> (5.2368, 110.7529) construction
  line L1405 (5.2368, 110.7529) -> (5.9084, 111.4245) construction
  line L1406 (5.9084, 111.4245) -> (5.9084, 112.2529) construction
  line L1407 (-3.1737, 117.4429) -> (1.8263, 117.4429)
  line L1408 (1.8263, 117.4429) -> (1.8263, 120.4429)
  line L1409 (1.8263, 120.4429) -> (-3.1737, 120.4429)
  line L1410 (-3.1737, 120.4429) -> (-3.1737, 117.4429)
  line L1411 (-43.3571, 66.8039) -> (-43.3571, 70.0912)
  line L1412 (-43.3571, 70.0912) -> (-59.3571, 70.0912)
  line L1413 (-59.3571, 70.0912) -> (-59.3571, 66.8039)
  line L1414 (-43.3571, 66.8039) -> (-22.8236, 66.8039)
  line L1415 (-22.8236, 66.8039) -> (-22.8236, 61.0912)
  line L1416 (-22.8236, 61.0912) -> (-82.3571, 61.0912)
  line L1417 (-82.3571, 61.0912) -> (-82.3571, 66.8039)
  line L1418 (-82.3571, 66.8039) -> (-59.3571, 66.8039)
  line L1419 (-16.3571, 117.4429) -> (-21.3571, 117.4429)
  line L1420 (-21.3571, 117.4429) -> (-21.3571, 120.4429)
  line L1421 (-21.3571, 120.4429) -> (-16.3571, 120.4429)
  line L1422 (-16.3571, 120.4429) -> (-16.3571, 117.4429)
  line L1423 (-16.3571, 58.7395) -> (-21.3571, 58.7395)
  line L1424 (-21.3571, 58.7395) -> (-21.3571, 55.7395)
  line L1425 (-21.3571, 55.7395) -> (-16.3571, 55.7395)
  line L1426 (-16.3571, 55.7395) -> (-16.3571, 58.7395)
  line L1427 (-100.3571, 85.0242) -> (-100.3571, 82.5913)
  line L1428 (-100.3571, 66.5242) -> (-83.849, 66.5242)
  line L1429 (-83.849, 66.5242) -> (-83.849, 82.5912)
  line L1430 (-83.849, 82.5912) -> (-100.3571, 82.5912)
  line L1431 (-100.3571, 85.0242) -> (-83.849, 85.0242)
  line L1432 (-83.849, 85.0242) -> (-83.849, 101.0911)
  line L1433 (-83.849, 101.0911) -> (-100.3571, 101.0911)
  line L1434 (-93.1735, 58.7395) -> (-88.1735, 58.7395)
  line L1435 (-88.1735, 58.7395) -> (-88.1735, 55.7395)
  line L1436 (-88.1735, 55.7395) -> (-93.1735, 55.7395)
  line L1437 (-93.1735, 55.7395) -> (-93.1735, 58.7395)
  line L1438 (-82.3571, 109.3785) -> (-22.8236, 109.3785)
  line L1439 (-22.8236, 109.3785) -> (-22.8236, 115.0911)
  line L1440 (-22.8236, 115.0911) -> (-82.3571, 115.0911)
  line L1441 (-82.3571, 115.0911) -> (-82.3571, 109.3785)
  line L1442 (-83.849, 66.5242) -> (-100.3571, 66.5242)
  line L1443 (-97.3571, 52.7395) -> (-86.2144, 52.7395) construction
  line L1444 (-100.3571, 66.5242) -> (-100.3571, 52.7395)
  line L1445 (-83.849, 66.5242) -> (-83.849, 82.5912)
  line L1446 (-83.849, 82.5912) -> (-100.3571, 82.5912)
  line L1447 (-100.3571, 82.5912) -> (-100.3571, 85.0242)
  line L1448 (-100.3571, 85.0242) -> (-83.849, 85.0242)
  line L1449 (-83.849, 85.0242) -> (-83.849, 101.0911)
  line L1450 (-83.849, 101.0911) -> (-100.3571, 101.0911)
  line L1451 (-100.3571, 101.0911) -> (-100.3571, 123.4429)
  line L1452 (-100.3571, 101.0911) -> (-75.9776, 101.0911) construction
  line L1453 (-97.3571, 123.4429) -> (-89.9825, 123.4429) construction
  line L1454 (-100.3571, 123.4429) -> (-13.3571, 123.4429)
  line L1455 (-100.3571, 52.7395) -> (-13.3571, 52.7395)
  line L1456 (-13.3571, 123.4429) -> (-13.3571, 52.7395)
  line L1457 (-16.3571, 120.4429) -> (-21.3571, 120.4429)
  line L1458 (-21.3571, 120.4429) -> (-21.3571, 117.4429)
  line L1459 (-21.3571, 117.4429) -> (-16.3571, 117.4429)
  line L1460 (-16.3571, 117.4429) -> (-16.3571, 120.4429)
  line L1461 (-16.3571, 58.7395) -> (-21.3571, 58.7395)
  line L1462 (-21.3571, 58.7395) -> (-21.3571, 55.7395)
  line L1463 (-21.3571, 55.7395) -> (-16.3571, 55.7395)
  line L1464 (-16.3571, 55.7395) -> (-16.3571, 58.7395)
  line L1465 (-34.6965, 76.0892) -> (-38.6965, 76.0892)
  line L1466 (-38.6965, 76.0892) -> (-38.6965, 73.0892)
  line L1467 (-38.6965, 73.0892) -> (-34.6965, 73.0892)
  line L1468 (-34.6965, 73.0892) -> (-34.6965, 76.0892)
  line L1469 (-88.1735, 120.4429) -> (-93.1735, 120.4429)
  line L1470 (-93.1735, 120.4429) -> (-93.1735, 117.4429)
  line L1471 (-93.1735, 117.4429) -> (-88.1735, 117.4429)
  line L1472 (-88.1735, 117.4429) -> (-88.1735, 120.4429)
  line L1473 (-89.2175, 113.1942) -> (-93.2175, 113.1942)
  line L1474 (-93.2175, 113.1942) -> (-93.2175, 110.1942)
  line L1475 (-93.2175, 110.1942) -> (-89.2175, 110.1942)
  line L1476 (-89.2175, 110.1942) -> (-89.2175, 113.1942)
  line L1477 (-89.2175, 106.1942) -> (-93.2175, 106.1942)
  line L1478 (-93.2175, 106.1942) -> (-93.2175, 103.1942)
  line L1479 (-93.2175, 103.1942) -> (-89.2175, 103.1942)
  line L1480 (-89.2175, 103.1942) -> (-89.2175, 106.1942)
  line L1481 (-88.1735, 58.7395) -> (-93.1735, 58.7395)
  line L1482 (-93.1735, 58.7395) -> (-93.1735, 55.7395)
  line L1483 (-93.1735, 55.7395) -> (-88.1735, 55.7395)
  line L1484 (-88.1735, 55.7395) -> (-88.1735, 58.7395)
  line L1485 (-22.8236, 115.0911) -> (-82.3571, 115.0911)
  line L1486 (-82.3571, 115.0911) -> (-82.3571, 109.3785)
  line L1487 (-82.3571, 109.3785) -> (-22.8236, 109.3785)
  line L1488 (-22.8236, 109.3785) -> (-22.8236, 115.0911)
  line L1489 (-22.8236, 61.0912) -> (-22.8236, 66.8039)
  line L1490 (-22.8236, 66.8039) -> (-43.3571, 66.8039)
  line L1491 (-43.3571, 66.8039) -> (-43.3571, 70.0912)
  line L1492 (-43.3571, 70.0912) -> (-59.3571, 70.0912)
  line L1493 (-59.3571, 70.0912) -> (-59.3571, 66.8039)
  line L1494 (-59.3571, 66.8039) -> (-82.3571, 66.8039)
  line L1495 (-82.3571, 66.8039) -> (-82.3571, 61.0912)
  line L1496 (-82.3571, 61.0912) -> (-22.8236, 61.0912)
  line L1497 (-18.0514, 67.168) -> (-21.0514, 67.168)
  circle A0 centre (-19.5514, 67.168) radius 1.5
  line L1498 (-84.0914, 112.2529) -> (-87.0914, 112.2529)
  circle A1 centre (-85.5914, 112.2529) radius 1.5
  line L1499 (-84.0914, 63.993) -> (-87.0914, 63.993)
  circle A2 centre (-85.5914, 63.993) radius 1.5
  point P0 (0, 0)
  dimension "d1" = 90
  constraints: 2628 end point, 17 parallel, 14 perpendicular, 13 horizontal, 8 collinear, 3 centre point, 3 coincident, 3 midpoint, 1 vertical, 102 other
  measures "d1" angle of L1452 L1451
extrude "Extrusion1" add sketch "Sketch1" along normal blind 3 contours L1428 L1429 L1430 L1427 L1431 L1432 L1433 L1169 L1168 L1167 L1166 L1165 L1164 L1163 L1162 L1161 L1160 L1159 L1158 L1157 L1156 L1155 L1154 L1153 L1152 L1151 L1150 L1149 L1148 L1147 L1146 L1145 L1144 L1143 L1142 L1141 L1140 L1139 L1138 L1137 L1136 L1135 L1134 L1133 L1132 L1131 L1130 L1129 L1128 L1127 L1126 L1125 L1124 L1123 L1122 L1121 L1120 L1119 L1118 L1117 L1116 L1115 L1114 L1113 L1112 L1111 L1110 L1109 L1108 L1107 L1106 L1105 L1104 L1103 L1102 L1101 L1100 L1099 L1098 L1097 L1096 L1095 L1094 L1093 L1092 L1091 L1090 L1089 L1088 L1087 L1086 L1085 L1084 L1083 L1082 L1081 L1080 L1079 L1078 L1077 L1076 L1075 L1074 L1073 L1072 L1071 L1070 L1069 L1068 L1067 L1066 L1065 L1064 L1063 L1062 L1061 L1060 L1059 L1058 L1057 L1056 L1055 L1054 L1053 L1052 L1051 L1050 L1049 L1048 L1047 L1046 L1045 L1044 L1043 L1042 L1041 L1040 L1039 L1038 L1037 L1036 L1035 L1034 L1033 L1032 L1031 L1030 L1029 L1028 L1027 L1026 L1025 L1024 L1023 L1022 L1021 L1020 L1019 L1018 L1017 L1016 L1015 L1014 L1013 L1012 L1011 L1010 L1009 L1008 L1007 L1006 L1005 L1004 L1003 L1002 L1001 L1000 L999 L998 L997 L996 L995 L994 L993 L992 L991 L990 L989 L988 L987 L986 L985 L984 L983 L982 L981 | L983 L984 L985 L986 L987 L988 L989 L990 L991 L992 L993 L994 L995 L996 L997 L998 L999 L1000 L1001 L1002 L1003 L1004 L1005 L1006 L1007 L1008 L1009 L1010 L1011 L1012 L1013 L1014 L1015 L1016 L1017 L1018 L1019 L1020 L1021 L1022 L1023 L1024 L1025 L1026 L1455 L1444 | L1030 L1031 L1032 L1033 L1034 L1035 L1036 L1037 L1038 L1039 L1040 L1041 L1042 L1043 L1044 L1045 L1046 L1047 L1048 L1049 L1050 L1051 L1052 L1053 L1054 L1055 L1056 L1057 L1058 L1059 L1060 L1061 L1062 L1063 L1064 L1065 L1066 L1067 L1068 L1069 L1070 L1071 L1072 L1073 L1456 L1455 | L1451 L1454 L1124 L1125 L1126 L1127 L1128 L1129 L1130 L1131 L1132 L1133 L1134 L1135 L1136 L1137 L1138 L1139 L1140 L1141 L1142 L1143 L1144 L1145 L1146 L1147 L1148 L1149 L1150 L1151 L1152 L1153 L1154 L1155 L1156 L1157 L1158 L1159 L1160 L1161 L1162 L1163 L1164 L1165 L1166 L1167 | L1077 L1078 L1079 L1080 L1081 L1082 L1083 L1084 L1085 L1086 L1087 L1088 L1089 L1090 L1091 L1092 L1093 L1094 L1095 L1096 L1097 L1098 L1099 L1100 L1101 L1102 L1103 L1104 L1105 L1106 L1107 L1108 L1109 L1110 L1111 L1112 L1113 L1114 L1115 L1116 L1117 L1118 L1119 L1120 L1454 L1456
fillet "Fillet1" radius 2 4 edges at (100.3571, 1.5, 123.4429) (13.3571, 1.5, 123.4429) (13.3571, 1.5, 52.7395) (100.3571, 1.5, 52.7395)
body "Solid1"
